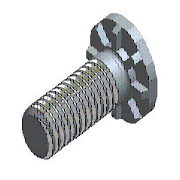
# Autodesk Inventor part: HFE-032-32 ZI
Saved by Autodesk Inventor 2024 (Build 280153000, 153)
## iProperties
IsCustomPart: 0
Created: 2023-01-19
Part Number: HFE-032-32 ZI
Material: Acero, carbono
Catalog Web Link: www.pemnet.com
Description: Espárragos PEM autorremachables HFE - Pulgadas
Vendor: PennEngineering®
Document SubType Name: Modeling
Standard: PEM
Designer: nesto
Manufacturer: PennEngineering®
Language: es-ES
Size Designation: HFE-032-32 ZI
Categories: <MemberInstance><Categories><Category DisplayName="Chapa metálica" InternalName="21944ee9-ad4d-44c9-9b1e-873eb7935d2a" Mnemonic="PEM"><Category DisplayName="Espárragos" InternalName="a2188e1b-484b-4305-8bf4-ec5c89769453" Mnemonic="pemStuds"><CategoryParameter DisplayName="Designación de serie de roscas" InternalName="03190524-7752-4605-8d0f-16dbfc9a5486" Mnemonic="thrserdsgn"/><CategoryParameter DisplayName="Diámetro del eje" InternalName="0798fc74-c739-4cf2-a250-69b5137ecf0b" Mnemonic="grpdia"/><CategoryParameter DisplayName="Hilos por unidad" InternalName="18c8b170-0f21-485b-b6b0-effffc919500" Mnemonic="thrperunit1"/><CategoryParameter DisplayName="Longitud nominal" InternalName="2b53957e-0aee-43be-b71a-49b2debece46" Mnemonic="nomlen"/><CategoryParameter DisplayName="Diámetro del agujero" InternalName="35967fbd-b0ea-4bd0-85e9-351650fbe2ab" Mnemonic="SMBHD"/><CategoryParameter DisplayName="Longitud del eje" InternalName="4f3018fe-66ab-43a1-8110-181b2668c0c7" Mnemonic="shnklen"/><CategoryParameter DisplayName="Designación de rosca" InternalName="5793e1d1-8c6a-4152-86f4-a921fb5aab9e" Mnemonic="thrdesign"/><CategoryParameter DisplayName="Grosor mínimo de chapa" InternalName="5b7d4485-c0aa-4517-a946-c6a5a269b27c" Mnemonic="SMBMIST"/><CategoryParameter DisplayName="Longitud de rosca" InternalName="6caf2edf-e86f-4e63-80ff-b45250d5ceee" Mnemonic="thrlen"/><CategoryParameter DisplayName="Clase de rosca" InternalName="91059bbb-7712-419d-8465-db77f0d91a13" Mnemonic="thrclss"/><CategoryParameter DisplayName="Tipo de rosca" InternalName="a3715b49-09e1-4797-90ad-cbfe5ea9b6ea" Mnemonic="thrtype"/><CategoryParameter DisplayName="Longitud asociada" InternalName="a513e428-3fb5-4a90-abdd-be9a7d5dab44" Mnemonic="grplen"/><CategoryParameter DisplayName="Diámetro nominal" InternalName="ca11677f-f1e9-4208-b7dc-003eed8d1536" Mnemonic="nomdia"/></Category></Category><Category DisplayName="TipoDatos" InternalName="23b78d0f-2648-40c6-8793-ca6db495c9e8" Mnemonic="DATATYPE"><CategoryParameter DisplayName="NombreVisualización" InternalName="05415f3d-3907-474b-a020-eb9d644f4cf3" Mnemonic="DISPLAYNAME"/><CategoryParameter DisplayName="Estándar" InternalName="0c0a119c-1e12-4c84-803f-101930972f5e" Mnemonic="STANDARD"/><CategoryParameter DisplayName="Descripción" InternalName="13903e3d-64b1-4950-80da-f627842ea37f" Mnemonic="DESCRIPTION"/><CategoryParameter DisplayName="Designación" InternalName="2675968c-4ce5-49e0-a4f5-552d29089031" Mnemonic="DESIGNATION"/><CategoryParameter DisplayName="Fila por defecto" InternalName="2af9ec52-faaa-4026-b378-f9fa4afca842" Mnemonic="DEFAULTROW"/><CategoryParameter DisplayName="Nombre de carpeta" InternalName="3f06958e-8713-4116-9be7-ed6184ecc97b" Mnemonic="FOLDERNAME"/><CategoryParameter DisplayName="Guid de revisión" InternalName="45a75005-10b1-4dfc-8d6d-dfe629f0b93c" Mnemonic="REVISIONGUID"/><CategoryParameter DisplayName="NombreArchivo" InternalName="8b46a4cc-9585-4fed-90c3-899f57e09a73" Mnemonic="FILENAME"/><CategoryParameter DisplayName="OrgEstand" InternalName="8f5914e1-4693-403f-8ab5-d37768198c9d" Mnemonic="STDSORG"/><CategoryParameter DisplayName="Versión de familia" InternalName="914462f6-6e19-4b14-ba84-155b9680b1d0" Mnemonic="FAMILYREVISION"/><CategoryParameter DisplayName="Revisión de Norma" InternalName="91d5a463-65c2-4fde-b823-3b7fea5e8e17" Mnemonic="STANDARDREVISION"/><CategoryParameter DisplayName="Revisión del miembro" InternalName="a65d44b9-392f-4f4f-857b-e4b3d54996fe" Mnemonic="MEMBERREVISION"/><CategoryParameter DisplayName="FormatoDelimitación" InternalName="bc51e27b-3422-4e78-93ef-cec197ddf230" Mnemonic="CLIPFORMAT"/><CategoryParameter DisplayName="Fabricante" InternalName="cd6c7a72-a28a-4e50-99a9-2c7f4e13e5ad" Mnemonic="MANUFACTURER"/><CategoryParameter DisplayName="NombreInterno" InternalName="cf1d0246-76d9-4b4a-8305-fa0409afb5c1" Mnemonic="INTERNALNAME"/><CategoryParameter DisplayName="EsMétrico" InternalName="e2385c5b-1ea4-4823-96a8-8de651266ec3" Mnemonic="ISMETRIC"/><Category DisplayName="Pieza" InternalName="c0e0b642-3bcb-4cc8-9e80-f96d35c4afa4" Mnemonic="PART"><CategoryParameter DisplayName="Número de pieza" InternalName="016b6077-bfbe-49bd-92c9-d8d59c39c941" Mnemonic="PARTNUMBER"/><CategoryParameter DisplayName="Referencia de almacén" InternalName="4dba7c1c-e26c-444e-836c-b08b433409a8" Mnemonic="STOCKNUMBER"/><CategoryParameter DisplayName="Clave de material" InternalName="5c9a8adb-dd2b-4535-b97f-0a94a95fe41f" Mnemonic="MATERIALKEY"/><CategoryParameter DisplayName="Material" InternalName="818a152a-d3c3-49ca-80ee-df7d91421b8e" Mnemonic="MATERIAL"/></Category></Category></Categories><FamilyTemplate Id="PEM Self-Clinching Studs HFE - Inch"><FamilyTemplateParameters><FamilyTemplateParameter ObjectType="kUserParameterObject" ValueType="xs:double" Id="1" ObjectReferenceKey="CH"/><FamilyTemplateParameter ObjectType="kUserParameterObject" ValueType="xs:double" Id="2" ObjectReferenceKey="D_"/><FamilyTemplateParameter ObjectType="kUserParameterObject" ValueType="xs:double" Id="3" ObjectReferenceKey="H_"/><FamilyTemplateParameter ObjectType="kUserParameterObject" ValueType="xs:double" Id="4" ObjectReferenceKey="H_Size"/><FamilyTemplateParameter ObjectType="kUserParameterObject" ValueType="xs:double" Id="5" ObjectReferenceKey="L"/><FamilyTemplateParameter ObjectType="kUserParameterObject" ValueType="xs:double" Id="7" ObjectReferenceKey="Max_Hole"/><FamilyTemplateParameter ObjectType="kUserParameterObject" ValueType="xs:double" Id="8" ObjectReferenceKey="Min_Dist"/><FamilyTemplateParameter ObjectType="kUserParameterObject" ValueType="xs:double" Id="9" ObjectReferenceKey="Min_Thick"/><FamilyTemplateParameter ObjectType="kUserParameterObject" ValueType="xs:double" Id="11" ObjectReferenceKey="R_"/><FamilyTemplateParameter ObjectType="kUserParameterObject" ValueType="xs:double" Id="12" ObjectReferenceKey="S_"/><FamilyTemplateParameter ObjectType="kUserParameterObject" ValueType="xs:double" Id="17" ObjectReferenceKey="th_"/><FamilyTemplateParameter ObjectType="kUserParameterObject" ValueType="xs:double" Id="18" ObjectReferenceKey="T_"/><FamilyTemplateParameter ObjectType="kPropertyObject" ValueType="xs:string" Id="100" ObjectReferenceKey="{32853F0F-3444-11d1-9E93-0060B03C1CA6}" SubObjectId="52"/><FamilyTemplateParameter ObjectType="kPropertyObject" ValueType="xs:string" Id="105" ObjectReferenceKey="{32853F0F-3444-11d1-9E93-0060B03C1CA6}" SubObjectId="5"/><FamilyTemplateParameter ObjectType="kPartComponentDefinitionObject" ValueType="xs:string" Id="110" SubObjectId="Material"/><FamilyTemplateParameter ObjectType="kThreadFeatureObject" ValueType="xs:structure" Id="300" ObjectReferenceKey="10020000100000005d210000000000008000000000000000" SubObjectId="ThreadInfo"><FamilyTemplateParameter ObjectType="" ValueType="xs:string" Id="301" SubObjectId="ThreadClass"/><FamilyTemplateParameter ObjectType="" ValueType="xs:string" Id="302" SubObjectId="ThreadDesignation"/><FamilyTemplateParameter ObjectType="" ValueType="xs:string" Id="303" SubObjectId="ThreadType"/><FamilyTemplateParameter ObjectType="" ValueType="xs:string" Id="304" SubObjectId="Pitch"/></FamilyTemplateParameter></FamilyTemplateParameters></FamilyTemplate><CategoryParameterMap><ParamToTemplateMap><ParamToTemplate CategoryParameter="//CategoryParameter[@InternalName='05415f3d-3907-474b-a020-eb9d644f4cf3']" ConstantValue="PEM Self-Clinching Studs HFE - Inch"/><ParamToTemplate CategoryParameter="//CategoryParameter[@InternalName='0c0a119c-1e12-4c84-803f-101930972f5e']" ConstantValue="PEM"/><ParamToTemplate CategoryParameter="//CategoryParameter[@InternalName='13903e3d-64b1-4950-80da-f627842ea37f']" ConstantValue="PEM Self-Clinching Studs HFE - Inch"/><ParamToTemplate CategoryParameter="//CategoryParameter[@InternalName='2af9ec52-faaa-4026-b378-f9fa4afca842']" ConstantValue="1"/><ParamToTemplate CategoryParameter="//CategoryParameter[@InternalName='3f06958e-8713-4116-9be7-ed6184ecc97b']" ConstantValue="PEM Self-Clinching Studs HFE - Inch"/><ParamToTemplate CategoryParameter="//CategoryParameter[@InternalName='45a75005-10b1-4dfc-8d6d-dfe629f0b93c']" ConstantValue="69ba914a-59b5-4449-a72e-0d8a9caf4376"/><ParamToTemplate CategoryParameter="//CategoryParameter[@InternalName='8f5914e1-4693-403f-8ab5-d37768198c9d']" TemplateParameter="101"/><ParamToTemplate CategoryParameter="//CategoryParameter[@InternalName='914462f6-6e19-4b14-ba84-155b9680b1d0']" ConstantValue="11"/><ParamToTemplate CategoryParameter="//CategoryParameter[@InternalName='91d5a463-65c2-4fde-b823-3b7fea5e8e17']" TemplateParameter="103"/><ParamToTemplate CategoryParameter="//CategoryParameter[@InternalName='bc51e27b-3422-4e78-93ef-cec197ddf230']" ConstantValue="CF_INVENTOR.STDPARTS"/><ParamToTemplate CategoryParameter="//CategoryParameter[@InternalName='cd6c7a72-a28a-4e50-99a9-2c7f4e13e5ad']" ConstantValue="PennEngineering®"/><ParamToTemplate CategoryParameter="//CategoryParameter[@InternalName='cf1d0246-76d9-4b4a-8305-fa0409afb5c1']" ConstantValue="3a6ddf92-385d-4ea5-b4a0-9fdba8f8ab75"/><ParamToTemplate CategoryParameter="//CategoryParameter[@InternalName='e2385c5b-1ea4-4823-96a8-8de651266ec3']" ConstantValue="false"/><ParamToTemplate CategoryParameter="//CategoryParameter[@InternalName='8b46a4cc-9585-4fed-90c3-899f57e09a73']" ConstantValue="HFE-032-32 ZI"/><ParamToTemplate CategoryParameter="//CategoryParameter[@InternalName='a65d44b9-392f-4f4f-857b-e4b3d54996fe']" ConstantValue="a69e0a88-54b7-4764-a6c9-954e8a2e98ac"/><ParamToTemplate CategoryParameter="//CategoryParameter[@InternalName='2675968c-4ce5-49e0-a4f5-552d29089031']" TemplateParameter="100"/><ParamToTemplate CategoryParameter="//CategoryParameter[@InternalName='ca11677f-f1e9-4208-b7dc-003eed8d1536']" TemplateParameter="2"/><ParamToTemplate CategoryParameter="//CategoryParameter[@InternalName='35967fbd-b0ea-4bd0-85e9-351650fbe2ab']" TemplateParameter="4"/><ParamToTemplate CategoryParameter="//CategoryParameter[@InternalName='2b53957e-0aee-43be-b71a-49b2debece46']" TemplateParameter="5"/><ParamToTemplate CategoryParameter="//CategoryParameter[@InternalName='6caf2edf-e86f-4e63-80ff-b45250d5ceee']" TemplateParameter="5"/><ParamToTemplate CategoryParameter="//CategoryParameter[@InternalName='818a152a-d3c3-49ca-80ee-df7d91421b8e']" TemplateParameter="110"/><ParamToTemplate CategoryParameter="//CategoryParameter[@InternalName='5b7d4485-c0aa-4517-a946-c6a5a269b27c']" TemplateParameter="9"/><ParamToTemplate CategoryParameter="//CategoryParameter[@InternalName='016b6077-bfbe-49bd-92c9-d8d59c39c941']" TemplateParameter="105"/><ParamToTemplate CategoryParameter="//CategoryParameter[@InternalName='4f3018fe-66ab-43a1-8110-181b2668c0c7']" TemplateParameter="12"/><ParamToTemplate CategoryParameter="//CategoryParameter[@InternalName='a513e428-3fb5-4a90-abdd-be9a7d5dab44']" TemplateParameter="18"/><ParamToTemplate CategoryParameter="//CategoryParameter[@InternalName='91059bbb-7712-419d-8465-db77f0d91a13']" TemplateParameter="301"/><ParamToTemplate CategoryParameter="//CategoryParameter[@InternalName='5793e1d1-8c6a-4152-86f4-a921fb5aab9e']" TemplateParameter="302"/><ParamToTemplate CategoryParameter="//CategoryParameter[@InternalName='a3715b49-09e1-4797-90ad-cbfe5ea9b6ea']" TemplateParameter="303"/></ParamToTemplateMap></CategoryParameterMap></MemberInstance>
Density: 7.85 g/cm^3
Appearance: Semipulido
Author: nesto
Autodesk Inventor part; units mm, degrees
ref_plane "YZ Plane" through (0, 0, 0) normal (1, 0, 0) x (0, 1, 0)
ref_plane "XZ Plane" through (0, 0, 0) normal (0, 1, 0) x (-1, 0, 0)
ref_plane "XY Plane" through (0, 0, 0) normal (0, 0, 1) x (1, 0, 0)
sketch "Sketch2" plane through (0, 0, 0) normal (0, 1, 0) x (-1, 0, 0)
  line L0 (0, 0) -> (4.5683, 0)
  line L1 (4.6699, 0.1016) -> (4.6699, 1.2192)
  line L2 (4.6699, 1.2192) -> (2.6162, 1.2192)
  line L3 (2.6162, 1.2192) -> (2.6162, 2.0828)
  line L4 (2.6162, 2.0828) -> (2.4232, 2.0828)
  line L5 (2.4232, 2.0828) -> (2.4232, 2.0787)
  line L6 (2.4232, 3.81) -> (2.413, 3.81)
  line L7 (2.413, 3.81) -> (2.413, 52.0192)
  line L8 (2.413, 52.0192) -> (0, 52.0192)
  line L9 (0, 52.0192) -> (0, 0)
  arc A0 (4.5683, 0) -> (4.6699, 0.1016) centre (4.5683, 0.1016) ccw
  arc A1 (2.4232, 2.794) -> (2.4232, 2.0787) centre (2.6162, 2.4364) ccw
  line L10 (2.4232, 2.794) -> (2.4232, 3.81)
  dimension "d0" = 4.826
  dimension "d1" = 9.3398
  dimension "d2" = 1.2192
  dimension "d3" = 50.8
  dimension "d4" = 2.5908
  dimension "d5" = 0.8636
  dimension "d6" = 4.8463
  dimension "d7" = 5.2324
  dimension "d8" = 0.1016
  dimension "d10" = 0.4064
  dimension "d12" = 0.7112
  constraints: 22 end point, 9 parallel, 4 point on circle, 2 centre point, 2 tangent, 1 collinear, 1 horizontal, 1 perpendicular, 1 point on line
  measures "d0" diameter of L7 L9
  measures "d1" diameter of L1 L9
  measures "d2" distance between parallel lines of L2 L0
  measures "d3" distance between parallel lines of L8 L2
  measures "d4" distance between parallel lines of L6 L2
  measures "d5" distance between parallel lines of L4 L2
  measures "d6" diameter of L5 L9
  measures "d7" diameter of L3 L9
  measures "d8" radius of A0
  measures "d10" radius of A1
  measures "d12" distance from line of L10.start L4
revolve "Revolución1" add sketch "Sketch2" angle 360 about axis through (0, 0, 52.0192) along (0, 0, -1)
thread "Rosca1" size "1/4" designation "1/4 - 18 NPT" standard "NPT for PVC Pipe and Fitting" length 15.113
chamfer "Chaflán1" distance 0.3048 angle 45 1 edges at (2.413, 0, 52.0192)
sketch "Sketch3" plane through (0, 0, 1.2192) normal (0, 0, 1) x (1, 0, 0)
  line L0 (0, 0) -> (0, 2.5843)
  circle A0 centre (0, 0) radius 2.6162 projected
  circle A1 centre (0, 0) radius 4.5339
  line L1 (-0.4001, 4.5162) -> (-0.4, 2.5854)
  line L2 (0.4001, 4.5162) -> (0.4, 2.5854)
  dimension "d18" = 9.0678
  dimension "d19" = 0.8001
  constraints: 6 end point, 4 point on circle, 2 parallel, 1 centre point, 1 coincident, 1 vertical, 1 other
  measures "d18" diameter of A1
  measures "d19" distance between parallel lines of L2 L1
extrude "Extrusión1" add sketch "Sketch3" along normal up to surface (0.8636 mm away) contours A0 L1 A1 L2 picked at (0.3113, 3.2381)
pattern_circular "Patrón circular1" count 8 over 360 about axis through (0, 0, -10) along (0, 0, 1) of "Extrusión1"
sketch "Sketch4" plane through (0, 0, 0) normal (0, 1, 0) x (-1, 0, 0)
  line L0 (-4.5162, 2.0828) -> (-2.5854, 2.0828) construction
  line L1 (-4.6699, 1.2192) -> (4.6699, 1.2192) construction
  line L2 (0, 0) -> (0, 2.462)
  line L3 (-4.5339, 1.2192) -> (-4.5339, 2.0828)
  line L4 (-4.5339, 2.0828) -> (-4.2196, 2.0828)
  line L5 (-4.2196, 2.0828) -> (-4.5339, 1.2192)
  dimension "d25" = 9.0678
  dimension "d26" = 20
  constraints: 8 end point, 2 point on line, 1 collinear, 1 parallel, 1 perpendicular
  measures "d25" diameter of L3 L2
  measures "d26" angle of L5 L3
revolve "Revolución2" cut sketch "Sketch4" angle 360 about axis through (0, 0, 0) along (0, 0, 1)
sketch "Sketch5" plane through (0, 0, 1.2192) normal (0, 0, 1) x (1, 0, 0)
  line L0 (4.5339, 1.878) -> (4.5339, -1.878) construction
  line L1 (4.5339, -1.878) -> (1.878, -4.5339) construction
  line L2 (1.878, -4.5339) -> (-1.878, -4.5339) construction
  line L3 (-1.878, -4.5339) -> (-4.5339, -1.878) construction
  line L4 (-4.5339, -1.878) -> (-4.5339, 1.878) construction
  line L5 (-4.5339, 1.878) -> (-1.878, 4.5339) construction
  line L6 (-1.1189, 4.5339) -> (1.1189, 4.5339)
  line L7 (1.878, 4.5339) -> (4.5339, 1.878) construction
  circle A0 centre (0, 0) radius 4.6699 projected
  dimension "d28" = 9.0678
  constraints: 16 end point, 2 point on circle, 1 coincident, 1 horizontal, 17 other
  measures "d28" distance between parallel lines of L2 L6
extrude "Extrusión2" cut sketch "Sketch5" against normal up to surface (1.2192 mm away) contours A0 L6 picked at (-0.1254, 4.5742)
pattern_circular "Patrón circular2" count 8 over 360 about axis through (0, 0, -10) along (0, 0, 1) of "Extrusión2"
sketch "Boceto6" plane through (0, 0, 52.0192) normal (0, 0, 1) x (1, 0, 0)
  point P0 (0, 0)
scale "Escala1" factors (6.665, 6.665, 6.665) then translate (0, 0, -157.2729) bodies 1
equation "\"d15\" = CH"
equation "\"d18\" = H_"
equation "\"d19\" = th_"
equation "\"d28\" = H_"
equation "\"d0\" = D_"
equation "\"d1\" = 1.03 * H_"
equation "\"d2\" = T_"
equation "\"d3\" = L"
equation "\"d4\" = S_"
equation "\"d5\" = 0.333333 * S_"
equation "\"d6\" = D_ + 0.2 * R_"
equation "\"d7\" = D_ + 4 * R_"
equation "\"d8\" = R_"
equation "\"d10\" = 4 * R_"
equation "\"d12\" = 7 * R_"
equation "\"d25\" = H_"
equation "\"L\" = 50.8"
equation "\"H_\" = 9.0678"
equation "\"S_\" = 2.5908"
equation "\"D_\" = 4.826"
equation "\"CH\" = 0.3048"
equation "\"R_\" = 0.1016"
equation "\"th_\" = 0.8001"
equation "\"T_\" = 1.2192"
equation "\"Min_Dist\" = 9.144"
equation "\"H_Size\" = 4.826"
equation "\"Min_Thick\" = 1.016"
equation "\"Max_Hole\" = 7.112"
body "Solid1"
